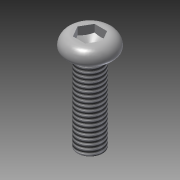
# Autodesk Inventor part: screw_M3_10_hex
Saved by Autodesk Inventor 2013 (Build 170138000, 138)
## iProperties
Shininess: 50.0
Created: 2012-07-28
Part Number: screw_M3_10_hex
Document SubType Name: Modeling
Designer: Noa Izumi
Material: Default
Density: 1 g/cm^3
Density: 0.0
Volumn: 0.0
Area: 0.0
PropertySet Name: Model Information
Control State: 0
Master: False
Checked Out: False
Author: Noa Izumi
Autodesk Inventor part; units mm, degrees
ref_plane "YZ Plane" through (0, 0, 0) normal (1, 0, 0) x (0, 1, 0)
ref_plane "XZ Plane" through (0, 0, 0) normal (0, 1, 0) x (-1, 0, 0)
ref_plane "XY Plane" through (0, 0, 0) normal (0, 0, 1) x (1, 0, 0)
sketch "Sketch1" plane through (0, 0, 0) normal (0, 0, 1) x (1, 0, 0)
  circle A0 centre (0, 0) radius 2.8
  dimension "d0" = 5.6
  constraints: 1 centre point
  measures "d0" diameter of A0
extrude "Extrusion1" add sketch "Sketch1" along normal blind 1.7
fillet "Fillet3" radius 0.5 1 edges at (-2.8, 0, 0)
fillet "Fillet4" radius 1.2 1 edges at (-2.8, 0, 1.7)
sketch "Sketch2" plane through (0, 0, 1.7) normal (0, 0, 1) x (1, 0, 0)
  line L0 (-0.75, -1.299) -> (0.75, -1.299)
  line L1 (0.75, -1.299) -> (1.5, 0)
  line L2 (1.5, 0) -> (0.75, 1.299)
  line L3 (0.75, 1.299) -> (-0.75, 1.299)
  line L4 (-0.75, 1.299) -> (-1.5, 0)
  line L5 (-1.5, 0) -> (-0.75, -1.299)
  dimension "d7" = 3
  constraints: 12 end point, 3 parallel
  measures "d7" distance of L4.end L1.end
extrude "Extrusion2" cut sketch "Sketch2" against normal blind 1.7
sketch "Sketch3" plane through (0, 0, 0) normal (0, 1, 0) x (-1, 0, 0)
  line L0 (0, 0) -> (1.5, 0)
  line L1 (2.3, 0) -> (-2.3, 0) projected
  line L2 (1.5, 0) -> (1.5, 0.8)
  line L3 (1.5, 0.8) -> (0, 0)
  line L4 (0, 0) -> (0, 2.432)
  dimension "d13" = 0
  dimension "d14" = 1.5
  dimension "d15" = 0.8
  constraints: 8 end point, 1 horizontal, 1 midpoint, 1 parallel, 1 perpendicular
  measures "d13" distance between parallel lines of L1 L0
  measures "d14" distance of L0.start L0.end
  measures "d15" distance of L0.end L2.end
revolve "Revolution2" add sketch "Sketch3" angle 360 about axis through (0, 0, 0) along (0, 0, 1)
sketch "Sketch4" plane through (0, 0, 0) normal (0, 0, -1) x (-1, 0, 0)
  circle A0 centre (0, 0) radius 2.3 projected
  circle A1 centre (0, 0) radius 1.5
  dimension "d18" = 3
  constraints: 1 centre point, 1 coincident
  measures "d18" diameter of A1
extrude "Extrusion3" add sketch "Sketch4" along normal blind 10 contours A1
thread "Thread1" size "M3x0.5" class "6g" standard "ANSI Metric M Profile" full length
